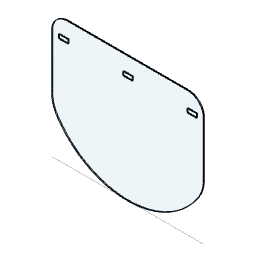
Face_Shield_V2 (Autodesk Fusion 360 design; units mm, degrees)
Autodesk Fusion 360 part; units mm, degrees
note: some values were not read from the file. Set by a fixed rule: which sketch regions a step uses.
sketch "Sketch1" plane through (0, 0, 0) normal (0, 0, 1) x (1, 0, 0)
  line L0 (25.4, 0) -> (219.964, 0)
  line L1 (245.364, -25.4) -> (245.364, -113.5343)
  line L2 (122.682, -203.2) -> (122.5934, -203.2)
  line L3 (0, -113.6694) -> (0, -25.4)
  arc A0 (8.3596, -141.588) -> (237.0568, -141.3732) centre (122.6377, -66.4123) ccw
  arc A1 (25.4, 0) -> (0, -25.4) centre (25.4, -25.4) ccw
  arc A2 (245.364, -25.4) -> (219.964, 0) centre (219.964, -25.4) ccw
  arc A3 (0, -113.6694) -> (8.3596, -141.588) centre (50.8, -113.6694) ccw
  arc A4 (237.0568, -141.3732) -> (245.364, -113.5343) centre (194.564, -113.5343) ccw
  line L4 (25.4, 0) -> (25.4, -25.4)
  line L5 (0, -25.4) -> (11.1506, -25.4)
  line L6 (11.1506, -25.4) -> (26.3906, -25.4)
  line L7 (26.3906, -25.4) -> (26.3906, -31.75)
  line L8 (26.3906, -31.75) -> (11.1506, -31.75)
  line L9 (11.1506, -31.75) -> (11.1506, -25.4)
  line L10 (122.682, 0) -> (122.682, -20.32) construction
  line L11 (234.2134, -25.4) -> (218.9734, -25.4)
  line L12 (218.9734, -25.4) -> (218.9734, -31.75)
  line L13 (218.9734, -31.75) -> (234.2134, -31.75)
  line L14 (234.2134, -31.75) -> (234.2134, -25.4)
  line L15 (122.682, 0) -> (122.682, -25.4)
  line L16 (122.682, -25.4) -> (130.302, -25.4)
  line L17 (130.302, -25.4) -> (130.302, -31.75)
  line L18 (130.302, -31.75) -> (115.062, -31.75)
  line L19 (115.062, -31.75) -> (115.062, -25.4)
  line L20 (115.062, -25.4) -> (122.682, -25.4)
  point P0 (245.364, 0)
  dimension "d1" = 245.364
  dimension "d3" = 25.4
  dimension "d4" = 50.8
  dimension "d5" = 11.1506
  dimension "d6" = 15.24
  dimension "d7" = 6.35
  dimension "d8" = 25.4
  dimension "d9" = 7.62
  dimension "d10" = 6.35
  dimension "d11" = 15.24
  dimension "d12" = 6.35
  constraint horizontal L0
  constraint vertical L1
  constraint horizontal L2
  constraint vertical L3
  constraint coincident origin L0
  constraint coincident origin L3
  constraint tangent L0 A1
  constraint tangent L3 A1
  constraint coincident P0 L0
  constraint coincident P0 L1
  constraint tangent L0 A2
  constraint tangent L1 A2
  constraint equal A1 A2
  constraint coincident A0 L2.end
  constraint coincident A0 L2.start
  constraint tangent A0 A3
  constraint tangent L3 A3
  constraint tangent A0 A4
  constraint tangent L1 A4
  constraint equal A3 A4
  constraint coincident A1.centre L4.end
  constraint perpendicular L3 L5
  constraint horizontal L6
  constraint vertical L7
  constraint horizontal L8
  constraint vertical L9
  constraint midpoint L0 L10.start
  constraint perpendicular L0 L10
  constraint symmetric L5.end L10 L11.start
  constraint symmetric L6.end L10 L11.end
  constraint symmetric L7.end L10 L12.end
  constraint symmetric L8.end L10 L13.end
  constraint perpendicular L0 L15
  constraint perpendicular L15 L16
  constraint perpendicular L0 L17
  constraint perpendicular L17 L18
  constraint perpendicular L18 L19
  measures "d1" distance of origin P0
  measures "d3" radius of A1
  measures "d4" radius of A3
  measures "d5" distance of L3.end L5.end
  measures "d6" distance of L5.end L6.end
  measures "d7" distance of L5.end L8.end
  measures "d8" distance of L10.start L15.end
  measures "d9" distance of L15.end L16.end
  measures "d10" distance of L16.end L17.end
  measures "d11" distance of L17.end L18.end
  measures "d12" distance of L18.end L19.end
extrude "Extrude1" add sketch "Sketch1" along normal blind 1.5875 draft 0.062 contours A1 L4 L5 L6 | L0 L1 L2 L3 A0 A2 A3 A4 L4 L5 L6 L7 L8 L9
sketch "Sketch2" plane through (0, 0, 1.5875) normal (0, 0, 1) x (1, 0, 0)
  line L0 (115.0637, -31.7483) -> (115.0637, -25.4017)
  line L1 (115.0637, -25.4017) -> (130.3003, -25.4017)
  line L2 (130.3003, -25.4017) -> (130.3003, -31.7483)
  line L3 (130.3003, -31.7483) -> (115.0637, -31.7483)
  line L4 (26.3889, -31.7483) -> (11.1523, -31.7483)
  line L5 (11.1523, -31.7483) -> (11.1523, -25.4017)
  line L6 (11.1523, -25.4017) -> (26.3889, -25.4017)
  line L7 (26.3889, -25.4017) -> (26.3889, -31.7483)
  line L8 (234.2117, -25.4017) -> (234.2117, -31.7483)
  line L9 (234.2117, -31.7483) -> (218.9751, -31.7483)
  line L10 (218.9751, -31.7483) -> (218.9751, -25.4017)
  line L11 (218.9751, -25.4017) -> (234.2117, -25.4017)
  arc A0 (-0.0017, -113.6694) -> (8.3581, -141.5889) centre (50.8, -113.6694) ccw
  arc A1 (8.3581, -141.5889) -> (237.0583, -141.3741) centre (122.6377, -66.4123) ccw
  arc A2 (237.0583, -141.3741) -> (245.3657, -113.5343) centre (194.564, -113.5343) ccw
  line L12 (245.3657, -113.5343) -> (245.3657, -25.4)
  arc A3 (245.3657, -25.4) -> (219.964, 0.0017) centre (219.964, -25.4) ccw
  line L13 (219.964, 0.0017) -> (25.4, 0.0017)
  arc A4 (25.4, 0.0017) -> (-0.0017, -25.4) centre (25.4, -25.4) ccw
  line L14 (-0.0017, -25.4) -> (-0.0017, -113.6694)
